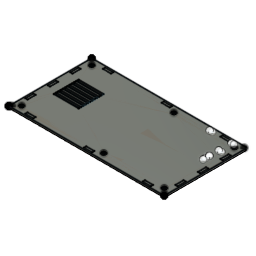
GBS 8200 Deckel v2 (Autodesk Fusion 360 design; units mm, degrees)
Autodesk Fusion 360 part; units mm, degrees
sketch "Skizze1" plane through (0, 0, 0) normal (0, 1, 0) x (1, 0, 0)
  line L0 (2, 0) -> (206, 0)
  line L1 (208, 2) -> (208, 109)
  line L2 (206, 111) -> (2, 111)
  line L3 (0, 109) -> (0, 2)
  circle A0 centre (8.575, 8.575) radius 1.5
  circle A1 centre (8.575, 102.425) radius 1.5
  circle A2 centre (199.425, 102.425) radius 1.5
  circle A3 centre (199.425, 8.575) radius 1.5
  line L4 (166.2, 106) -> (162.8, 106)
  line L5 (192, 106) -> (195.4, 106)
  line L6 (195.4, 89) -> (192, 89)
  line L7 (192, 68) -> (192, 76.4)
  line L8 (192, 76.4) -> (192, 71.4)
  line L9 (16.5, 77) -> (49.5, 77)
  line L10 (49.5, 77) -> (49.5, 44)
  line L11 (49.5, 44) -> (16.5, 44)
  line L12 (16.5, 44) -> (16.5, 77)
  line L13 (16.5, 77) -> (49.5, 77)
  line L14 (49.5, 77) -> (49.5, 74)
  line L15 (49.5, 74) -> (16.5, 74)
  line L16 (16.5, 74) -> (16.5, 77)
  line L17 (16.5, 74) -> (49.5, 74)
  line L18 (49.5, 74) -> (49.5, 71)
  line L19 (49.5, 71) -> (16.5, 71)
  line L20 (16.5, 71) -> (16.5, 74)
  line L21 (16.5, 71) -> (49.5, 71)
  line L22 (49.5, 71) -> (49.5, 68)
  line L23 (49.5, 68) -> (16.5, 68)
  line L24 (16.5, 68) -> (16.5, 71)
  line L25 (16.5, 68) -> (49.5, 68)
  line L26 (49.5, 68) -> (49.5, 65)
  line L27 (49.5, 65) -> (16.5, 65)
  line L28 (16.5, 65) -> (16.5, 68)
  line L29 (16.5, 65) -> (49.5, 65)
  line L30 (49.5, 65) -> (49.5, 62)
  line L31 (49.5, 62) -> (16.5, 62)
  line L32 (16.5, 62) -> (16.5, 65)
  line L33 (16.5, 62) -> (49.5, 62)
  line L34 (49.5, 62) -> (49.5, 59)
  line L35 (49.5, 59) -> (16.5, 59)
  line L36 (16.5, 59) -> (16.5, 62)
  line L37 (16.5, 59) -> (49.5, 59)
  line L38 (49.5, 59) -> (49.5, 56)
  line L39 (49.5, 56) -> (16.5, 56)
  line L40 (16.5, 56) -> (16.5, 59)
  line L41 (16.5, 56) -> (49.5, 56)
  line L42 (49.5, 56) -> (49.5, 53)
  line L43 (49.5, 53) -> (16.5, 53)
  line L44 (16.5, 53) -> (16.5, 56)
  line L45 (16.5, 53) -> (49.5, 53)
  line L46 (49.5, 53) -> (49.5, 50)
  line L47 (49.5, 50) -> (16.5, 50)
  line L48 (16.5, 50) -> (16.5, 53)
  line L49 (16.5, 50) -> (49.5, 50)
  line L50 (49.5, 50) -> (49.5, 47)
  line L51 (49.5, 47) -> (16.5, 47)
  line L52 (16.5, 47) -> (16.5, 50)
  line L53 (16.5, 47) -> (49.5, 47)
  line L54 (49.5, 47) -> (49.5, 44)
  line L55 (49.5, 44) -> (16.5, 44)
  line L56 (16.5, 44) -> (16.5, 47)
  line L57 (20, 109) -> (30.8, 109)
  line L58 (30.8, 109) -> (30.8, 106)
  line L59 (30.8, 106) -> (20, 106)
  line L60 (20, 106) -> (20, 109)
  line L61 (2, 91) -> (5, 91)
  line L62 (5, 91) -> (5, 80.2)
  line L63 (5, 80.2) -> (2, 80.2)
  line L64 (2, 80.2) -> (2, 91)
  line L65 (2, 30.8) -> (5, 30.8)
  line L66 (5, 30.8) -> (5, 20)
  line L67 (5, 20) -> (2, 20)
  line L68 (2, 20) -> (2, 30.8)
  line L69 (20, 5) -> (30.8, 5)
  line L70 (30.8, 5) -> (30.8, 2)
  line L71 (30.8, 2) -> (20, 2)
  line L72 (20, 2) -> (20, 5)
  line L73 (177.2, 5) -> (188, 5)
  line L74 (188, 5) -> (188, 2)
  line L75 (188, 2) -> (177.2, 2)
  line L76 (177.2, 2) -> (177.2, 5)
  line L77 (203, 30.8) -> (206, 30.8)
  line L78 (206, 30.8) -> (206, 20)
  line L79 (206, 20) -> (203, 20)
  line L80 (203, 20) -> (203, 30.8)
  line L81 (177.2, 109) -> (188, 109)
  line L82 (188, 109) -> (188, 106)
  line L83 (188, 106) -> (177.2, 106)
  line L84 (177.2, 106) -> (177.2, 109)
  line L85 (203, 91) -> (206, 91)
  line L86 (206, 91) -> (206, 80.2)
  line L87 (206, 80.2) -> (203, 80.2)
  line L88 (203, 80.2) -> (203, 91)
  line L89 (98.6, 5) -> (109.4, 5)
  line L90 (109.4, 5) -> (109.4, 2)
  line L91 (109.4, 2) -> (98.6, 2)
  line L92 (98.6, 2) -> (98.6, 5)
  line L93 (98.6, 109) -> (109.4, 109)
  line L94 (109.4, 109) -> (109.4, 106)
  line L95 (109.4, 106) -> (98.6, 106)
  line L96 (98.6, 106) -> (98.6, 109)
  line L97 (203, 60.9) -> (206, 60.9)
  line L98 (206, 60.9) -> (206, 50.1)
  line L99 (206, 50.1) -> (203, 50.1)
  line L100 (203, 50.1) -> (203, 60.9)
  line L101 (2, 60.9) -> (5, 60.9)
  line L102 (5, 60.9) -> (5, 50.1)
  line L103 (5, 50.1) -> (2, 50.1)
  line L104 (2, 50.1) -> (2, 60.9)
  arc A4 (2, 111) -> (0, 109) centre (2, 109) ccw
  arc A5 (0, 2) -> (2, 0) centre (2, 2) ccw
  arc A6 (206, 0) -> (208, 2) centre (206, 2) ccw
  arc A7 (208, 109) -> (206, 111) centre (206, 109) ccw
  circle A8 centre (118.425, 8.575) radius 1.5
  circle A9 centre (118.425, 102.425) radius 1.5
  point P0 (208, 0)
  point P1 (0, 111)
  dimension "d1" = 208
  dimension "d2" = 111
  dimension "d3" = 3
  dimension "d4" = 8.575
  dimension "d5" = 8.575
  dimension "d6" = 3
  dimension "d7" = 8.575
  dimension "d8" = 8.575
  dimension "d9" = 3
  dimension "d10" = 8.575
  dimension "d11" = 8.575
  dimension "d12" = 3
  dimension "d13" = 8.575
  dimension "d14" = 8.575
  dimension "d44" = 25.8
  dimension "d48" = 3.4
  dimension "d49" = 3.4
  dimension "d50" = 17
  dimension "d60" = 33
  dimension "d61" = 33
  dimension "d62" = 34
  dimension "d63" = 16.5
  dimension "d64" = 3
  dimension "d65" = 33
  dimension "d66" = 3
  dimension "d67" = 3
  dimension "d68" = 3
  dimension "d69" = 3
  dimension "d70" = 3
  dimension "d71" = 3
  dimension "d72" = 3
  dimension "d73" = 3
  dimension "d74" = 3
  dimension "d75" = 10.8
  dimension "d76" = 3
  dimension "d77" = 20
  dimension "d78" = 2
  dimension "d79" = 3
  dimension "d80" = 10.8
  dimension "d81" = 2
  dimension "d82" = 20
  dimension "d83" = 3
  dimension "d84" = 10.8
  dimension "d85" = 2
  dimension "d86" = 20
  dimension "d87" = 10.8
  dimension "d88" = 3
  dimension "d89" = 2
  dimension "d90" = 20
  dimension "d91" = 10.8
  dimension "d92" = 3
  dimension "d93" = 2
  dimension "d94" = 20
  dimension "d95" = 3
  dimension "d96" = 10.8
  dimension "d97" = 2
  dimension "d98" = 20
  dimension "d99" = 10.8
  dimension "d100" = 3
  dimension "d101" = 2
  dimension "d102" = 20
  dimension "d103" = 3
  dimension "d104" = 10.8
  dimension "d105" = 2
  dimension "d106" = 20
  dimension "d107" = 10.8
  dimension "d108" = 3
  dimension "d109" = 2
  dimension "d110" = 98.6
  dimension "d111" = 10.8
  dimension "d112" = 3
  dimension "d113" = 2
  dimension "d114" = 98.6
  dimension "d115" = 3
  dimension "d116" = 10.8
  dimension "d117" = 2
  dimension "d118" = 50.1
  dimension "d119" = 3
  dimension "d120" = 10.8
  dimension "d121" = 2
  dimension "d122" = 50.1
  dimension "d123" = 2
  dimension "d124" = 2
  dimension "d125" = 2
  dimension "d126" = 2
  dimension "d160" = 3
  dimension "d161" = 109.85
  dimension "d162" = 8.575
  dimension "d163" = 3
  dimension "d164" = 8.575
  dimension "d165" = 109.85
  constraint horizontal L0
  constraint vertical L1
  constraint horizontal L2
  constraint vertical L3
  constraint horizontal L4
  constraint horizontal L5
  constraint horizontal L6
  constraint vertical L7
  constraint vertical L8
  constraint horizontal L9
  constraint vertical L10
  constraint horizontal L11
  constraint vertical L12
  constraint horizontal L13
  constraint vertical L14
  constraint horizontal L15
  constraint vertical L16
  constraint horizontal L17
  constraint vertical L18
  constraint horizontal L19
  constraint vertical L20
  constraint horizontal L21
  constraint vertical L22
  constraint horizontal L23
  constraint vertical L24
  constraint horizontal L25
  constraint vertical L26
  constraint horizontal L27
  constraint vertical L28
  constraint horizontal L29
  constraint vertical L30
  constraint horizontal L31
  constraint vertical L32
  constraint horizontal L33
  constraint vertical L34
  constraint horizontal L35
  constraint vertical L36
  constraint horizontal L37
  constraint vertical L38
  constraint horizontal L39
  constraint vertical L40
  constraint horizontal L41
  constraint vertical L42
  constraint horizontal L43
  constraint vertical L44
  constraint horizontal L45
  constraint vertical L46
  constraint horizontal L47
  constraint vertical L48
  constraint horizontal L49
  constraint vertical L50
  constraint horizontal L51
  constraint vertical L52
  constraint horizontal L53
  constraint vertical L54
  constraint horizontal L55
  constraint vertical L56
  constraint horizontal L57
  constraint vertical L58
  constraint horizontal L59
  constraint vertical L60
  constraint horizontal L61
  constraint vertical L62
  constraint horizontal L63
  constraint vertical L64
  constraint horizontal L65
  constraint vertical L66
  constraint horizontal L67
  constraint vertical L68
  constraint horizontal L69
  constraint vertical L70
  constraint horizontal L71
  constraint vertical L72
  constraint horizontal L73
  constraint vertical L74
  constraint horizontal L75
  constraint vertical L76
  constraint horizontal L77
  constraint vertical L78
  constraint horizontal L79
  constraint vertical L80
  constraint horizontal L81
  constraint vertical L82
  constraint horizontal L83
  constraint vertical L84
  constraint horizontal L85
  constraint vertical L86
  constraint horizontal L87
  constraint vertical L88
  constraint horizontal L89
  constraint vertical L90
  constraint horizontal L91
  constraint vertical L92
  constraint horizontal L93
  constraint vertical L94
  constraint horizontal L95
  constraint vertical L96
  constraint horizontal L97
  constraint vertical L98
  constraint horizontal L99
  constraint vertical L100
  constraint horizontal L101
  constraint vertical L102
  constraint horizontal L103
  constraint vertical L104
  constraint coincident P1 L2
  constraint coincident P1 L3
  constraint tangent L2 A4
  constraint tangent L3 A4
  constraint coincident origin L3
  constraint coincident origin L0
  constraint tangent L3 A5
  constraint tangent L0 A5
  constraint coincident P0 L1
  constraint coincident P0 L0
  constraint tangent L1 A6
  constraint tangent L0 A6
  constraint tangent L2 A7
  constraint tangent L1 A7
  measures "d1" distance of origin P0
  measures "d2" distance of origin P1
  measures "d3" diameter of A0
  measures "d4" distance of L3 A0.centre
  measures "d5" distance of L0 A0.centre
  measures "d6" diameter of A1
  measures "d7" distance of L2 A1.centre
  measures "d8" distance of L3 A1.centre
  measures "d9" diameter of A2
  measures "d10" distance of L1 A2.centre
  measures "d11" distance of L2 A2.centre
  measures "d12" diameter of A3
  measures "d13" distance of L1 A3.centre
  measures "d14" distance of L0 A3.centre
  measures "d44" distance of L4.start L5.start
  measures "d48" distance of L4.start L4.end
  measures "d49" distance of L5.start L5.end
  measures "d50" distance of L5.end L6.start
  measures "d60" distance of L9.start L9.end
  measures "d61" distance of L9.start L11.end
  measures "d62" distance of L2 L9
  measures "d63" distance of L3 L12
  measures "d64" distance of L9.start L15.end
  measures "d65" distance of L15.end L14.end
  measures "d66" distance of L15.end L19.end
  measures "d67" distance of L19.end L23.end
  measures "d68" distance of L23.end L27.end
  measures "d69" distance of L27.end L31.end
  measures "d70" distance of L31.end L35.end
  measures "d71" distance of L35.end L39.end
  measures "d72" distance of L39.end L43.end
  measures "d73" distance of L43.end L47.end
  measures "d74" distance of L47.end L51.end
  measures "d75" distance of L57.start L57.end
  measures "d76" distance of L57.start L59.end
  measures "d77" distance of L3 L60
  measures "d78" distance of L2 L57
  measures "d79" distance of L61.start L61.end
  measures "d80" distance of L61.start L63.end
  measures "d81" distance of L3 L64
  measures "d82" distance of L2 L61.end
  measures "d83" distance of L65.start L65.end
  measures "d84" distance of L65.start L67.end
  measures "d85" distance of L3 L68
  measures "d86" distance of L0 L67.end
  measures "d87" distance of L69.start L69.end
  measures "d88" distance of L69.start L71.end
  measures "d89" distance of L0 L70.end
  measures "d90" distance of L3 L69.start
  measures "d91" distance of L73.start L73.end
  measures "d92" distance of L73.start L75.end
  measures "d93" distance of L0 L74.end
  measures "d94" distance of L1 L74.end
  measures "d95" distance of L77.start L77.end
  measures "d96" distance of L77.start L79.end
  measures "d97" distance of L1 L78
  measures "d98" distance of L0 L79.end
  measures "d99" distance of L81.start L81.end
  measures "d100" distance of L81.start L83.end
  measures "d101" distance of L2 L81
  measures "d102" distance of L1 L82
  measures "d103" distance of L85.start L85.end
  measures "d104" distance of L85.start L87.end
  measures "d105" distance of L1 L86
  measures "d106" distance of L2 L85
  measures "d107" distance of L89.start L89.end
  measures "d108" distance of L89.start L91.end
  measures "d109" distance of L0 L91
  measures "d110" distance of L3 L91.end
  measures "d111" distance of L93.start L93.end
  measures "d112" distance of L93.start L95.end
  measures "d113" distance of L2 L93
  measures "d114" distance of L3 L95.end
  measures "d115" distance of L97.start L97.end
  measures "d116" distance of L97.start L99.end
  measures "d117" distance of L1 L98
  measures "d118" distance of L2 L97
  measures "d119" distance of L101.start L101.end
  measures "d120" distance of L101.start L103.end
  measures "d121" distance of L3 L104
  measures "d122" distance of L2 L101.end
  measures "d123" radius of A4
  measures "d124" radius of A5
  measures "d125" radius of A6
  measures "d126" radius of A7
  measures "d160" diameter of A8
  measures "d161" horizontal distance of A0.centre A8.centre
  measures "d162" distance of L0 A8.centre
  measures "d163" diameter of A9
  measures "d164" distance of L2 A9.centre
  measures "d165" distance of A1.centre A9.centre
extrude "Extrusion11" add sketch "Skizze1" against normal blind 2.4 contours L0 L1 L2 L3 A4 A5 A6 A7 | L10 L12 L15 L17 L18 L19 L20 L21 | L10 L12 L23 L25 L26 L27 L28 L29 | L10 L12 L31 L33 L34 L35 L36 L37 | L10 L12 L39 L41 L42 L43 L44 L45 | L10 L12 L47 L49 L50 L51 L52 L53
extrude "Extrusion12" add sketch "Skizze1" against normal blind 0.6 contours L57 L58 L59 L60 | L61 L62 L63 L64 | L65 L66 L67 L68 | L69 L70 L71 L72 | L73 L74 L75 L76 | L77 L78 L79 L80 | L81 L82 L83 L84 | L85 L86 L87 L88 | L89 L90 L91 L92 | L93 L94 L95 L96 | L97 L98 L99 L100 | L101 L102 L103 L104
hole "Bohrung5" at (8.575, 0, -8.575) direction (0, -1, 0) diameter 6 depth 0.9 tip angle 180
hole "Bohrung6" at (8.575, 0, -102.425) direction (0, -1, 0) diameter 6 depth 0.9 tip angle 180
hole "Bohrung7" at (118.425, 0, -102.425) direction (0, -1, 0) diameter 6 depth 0.9 tip angle 180
hole "Bohrung8" at (118.425, 0, -8.575) direction (0, -1, 0) diameter 6 depth 0.9 tip angle 180
hole "Bohrung9" at (199.425, 0, -102.425) direction (0, -1, 0) diameter 6 depth 0.9 tip angle 180
hole "Bohrung10" at (199.425, 0, -8.575) direction (0, -1, 0) diameter 6 depth 0.9 tip angle 180
